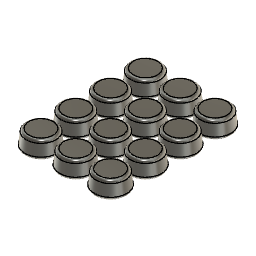
button cap v5 (Autodesk Fusion 360 design; units mm, degrees)
Autodesk Fusion 360 part; units mm, degrees
sketch "Sketch1" plane through (0, 0, 0) normal (0, 0, 1) x (1, 0, 0)
  circle A0 centre (0, 0) radius 1.6
  circle A1 centre (0, 0) radius 1.8
  circle A2 centre (0, 0) radius 5
  circle A3 centre (0, 0) radius 5.7
  dimension "d1" = 3.2
  dimension "d3" = 10
  dimension "d4" = 11.4
  dimension "d15" = 0.2
  constraint coincident A0.centre A1.centre
  constraint concentric A0 A3
  measures "d1" diameter of A0
  measures "d3" diameter of A2
  measures "d4" diameter of A3
  measures "d15" distance of A0 A1
ref_plane "WorkPlane1" through (0, 0, 5.8) normal (0, 0, 1) x (1, 0, 0)
sketch "Sketch2" plane through (0, 0, 5.8) normal (0, 0, 1) x (1, 0, 0)
  circle A0 centre (0, 0) radius 5
loft "Loft1" add profiles "Sketch1", "Sketch2" section 1 contours A2 | A3 section 2 makes body 1
ref_plane "WorkPlane2" through (0, 0, 4.4) normal (0, 0, 1) x (1, 0, 0)
sketch "Sketch3" plane through (0, 0, 4.4) normal (0, 0, 1) x (1, 0, 0)
  circle A0 centre (0, 0) radius 1.6
loft "Loft2" cut profiles "Sketch1", "Sketch3" section 1 contours A0 | A1 section 2 bodies 1
fillet "Fillet1" radius 1 1 edges at (-4.6616, 1.8081, 5.8) on bodies 1
fillet "Fillet1" radius 1 1 edges at (-5.3143, -2.0612, 0) on bodies 1
pattern_linear "R-Pattern1" count 4 spacing 12 along (0, 1, 0) count 3 spacing 12 along (1, 0, 0) of bodies 1 makes body 2 at (-0.4082, 6.5523, 1.9643) makes body 3 at (2.7315, 19.269, 1.9643) makes body 4 at (5.4019, 36.8142, 1.9643) makes body 5 at (10.0042, -5.0853, 1.9643) makes body 6 at (16.0046, 8.2843, 1.9643) makes body 7 at (14.7315, 28.731, 1.9643) makes body 8 at (17.4019, 36.8142, 1.9643) makes body 9 at (22.0042, -5.0853, 1.9643) makes body 10 at (22.0042, 6.9147, 1.9643) makes body 11 at (26.7315, 19.269, 1.9643) makes body 12 at (29.4019, 36.8142, 1.9643)
named bodies: "button cap", "button cap (1)", "button cap (2)", "button cap (3)", "button cap (4)", "button cap (5)", "button cap (6)", "button cap (7)", "button cap (8)", "button cap (9)", "button cap (10)", "button cap (11)"
